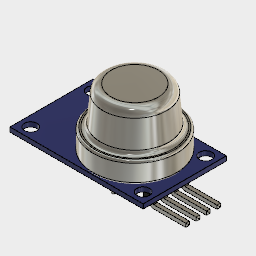
MQ135_sensor (Autodesk Fusion 360 design; units mm, degrees)
Autodesk Fusion 360 part; units mm, degrees
note: some values were not read from the file. Chosen so that the rebuilt part matches the saved one: which bodies a step acts on. Set by a fixed rule: which sketch regions a step uses.
sketch "Sketch1" plane through (0, 0, 0) normal (0, 0, 1) x (1, 0, 0)
  line L0 (-18.5, 15.5) -> (13.5, 15.5)
  line L1 (13.5, 15.5) -> (13.5, -4.5)
  line L2 (13.5, -4.5) -> (-18.5, -4.5)
  line L3 (-18.5, -4.5) -> (-18.5, 15.5)
  line L4 (-18.5, 5.5) -> (13.5, 5.5) construction
  line L5 (-2.5, 15.5) -> (-2.5, -4.5) construction
  line L6 (-16, 13) -> (11, 13) construction
  line L7 (11, 13) -> (11, -2) construction
  line L8 (11, -2) -> (-16, -2) construction
  line L9 (-16, -2) -> (-16, 13) construction
  circle A0 centre (-16, 13) radius 1.5
  circle A1 centre (-16, -2) radius 1.5
  circle A2 centre (11, 13) radius 1.5
  circle A3 centre (11, -2) radius 1.5
  line L10 (11.5, 19) -> (11.5, -9) construction
  circle A4 centre (1.5, 5.5) radius 10
  dimension "d1" = 20
  dimension "d2" = 32
  dimension "d3" = 27
  dimension "d4" = 15
  dimension "d5" = 3
  dimension "d6" = 3
  dimension "d7" = 3
  dimension "d8" = 3
  dimension "d9" = 2
  dimension "d10" = 20
  measures "d1" distance of L0.start L2.end
  measures "d2" distance of L0.start L0.end
  measures "d3" distance of L6.start L6.end
  measures "d4" distance of L6.start L8.end
  measures "d5" diameter of A0
  measures "d6" diameter of A1
  measures "d7" diameter of A2
  measures "d8" diameter of A3
  measures "d9" distance of L1 L10
  measures "d10" diameter of A4
extrude "Extrude1" add sketch "Sketch1" against normal blind 1.1 makes body 1
extrude "Extrude2" add sketch "Sketch1" along normal blind 5 separate body contours A4 makes body 2
sketch "Sketch2" plane through (0, 0, 5) normal (0, 0, 1) x (-1, 0, 0)
  circle A0 centre (-1.5, -5.5) radius 10
  circle A1 centre (-1.5, -5.5) radius 8.25
  dimension "d15" = 16.5
  measures "d15" diameter of A1
extrude "Extrude3" add sketch "Sketch2" along normal blind 9 draft -5 contours A1 bodies 2
fillet "Fillet1" radius 2 1 edges at (8.4576, 2.8014, 14) on bodies 2
fillet "Fillet2" radius 1 1 edges at (9.1917, 2.5167, 5) on bodies 2
fillet "Fillet3" radius 0.5 2 edges at (-7.8233, 1.8838, 5) (-7.8233, 1.8838, 0) on bodies 2
sketch "Sketch3" plane through (0, 0, -1.1) normal (0, 0, -1) x (1, 0, 0)
  circle A0 centre (11, 2) radius 1.5
  circle A1 centre (11, -13) radius 1.5
  circle A2 centre (-16, 2) radius 1.5
  circle A3 centre (-16, -13) radius 1.5
  line L0 (13.5, 4.5) -> (-18.5, 4.5)
  line L1 (-18.5, 4.5) -> (-18.5, -15.5)
  line L2 (-18.5, -15.5) -> (13.5, -15.5)
  line L3 (13.5, -15.5) -> (13.5, 4.5)
  line L4 (-12, -20) -> (-12, 7) construction
  line L5 (-18.5, 4.5) -> (-18.5, -15.5)
  line L6 (-12, -15) -> (-5, -15)
  line L7 (-5, -15) -> (-5, -8)
  line L8 (-5, -8) -> (-12, -8)
  line L9 (-12, -8) -> (-12, -15)
  line L10 (1.5, -19) -> (1.5, 10) construction
  line L11 (13.5, -15.5) -> (13.5, 4.5)
  circle A4 centre (1.5, -5.5) radius 5
  circle A5 centre (1.5, -10.5) radius 0.5
  circle A6 centre (5.0355, -9.0355) radius 0.5
  circle A7 centre (5.0355, -1.9645) radius 0.5
  circle A8 centre (1.5, -0.5) radius 0.5
  circle A9 centre (-2.0355, -1.9645) radius 0.5
  circle A10 centre (-2.0355, -9.0355) radius 0.5
  line L12 (11, -10.5) -> (8.5, -10.5)
  line L13 (8.5, -10.5) -> (8.5, -0.5)
  line L14 (8.5, -0.5) -> (11, -0.5)
  line L15 (11, -0.5) -> (11, -10.5)
  line L16 (11, -13) -> (11, 2)
  line L17 (-18.5, -5.5) -> (13.5, -5.5)
  point P0 (1.5, -5.5)
  dimension "d21" = 6.5
  dimension "d22" = 7
  dimension "d23" = 7
  dimension "d24" = 12
  dimension "d25" = 10
  dimension "d26" = 1
  dimension "d28" = 360
  dimension "d29" = 10
  dimension "d30" = 2.5
  measures "d21" distance of L4 L5
  measures "d22" distance of L6.start L8.end
  measures "d23" distance of L6.start L6.end
  measures "d24" distance of L10 L11
  measures "d25" diameter of A4
  measures "d26" diameter of A5
  measures "d29" distance of L12.start L14.end
  measures "d30" distance of L12.start L12.end
extrude "Extrude4" add sketch "Sketch3" along normal blind 5 separate body contours L6 L7 L8 L9 makes body 3
extrude "Extrude5" add sketch "Sketch3" along normal blind 5 separate body contours A4 A9 | A4 A9 | A4 A10 | A4 A10 | A4 A7 | A4 A7 | A4 A6 | A4 A6 | A4 A8 | A4 A8 | A4 A5 | A4 A5 makes body 4 at (-2.5349, 9.0106, -4.4333) makes body 5 at (5.533, 2.0142, -2.7667) makes body 6 at (1.9975, 10.4502, -4.4333) makes body 7 at (-1.538, 2.0142, -2.7667) makes body 8 at (1.9975, 0.5498, -2.7667) makes body 9 at (5.533, 8.9857, -4.4333)
combine "Combine1" operation add target body 9 tool bodies 8 7 6 5 4 makes body 10 at (-1.538, 2.0142, -2.7667) makes body 11 at (5.533, 2.0142, -2.7667) makes body 12 at (1.9975, 0.5498, -2.7667) makes body 13 at (1.9975, 10.4502, -4.4333) makes body 14 at (-2.5349, 9.0106, -4.4333)
extrude "Extrude6" add sketch "Sketch3" along normal blind 2.5 separate body contours L13 L14 L15 L16 L17 | L12 L13 L15 L16 L17 makes body 15
sketch "Sketch6" plane through (0, 0, -6.1) normal (0, 0, -1) x (1, 0, 0)
  line L0 (-12, -8) -> (-12, -15)
  line L1 (-12, -15) -> (-5, -15)
  line L2 (-5, -15) -> (-5, -8)
  line L3 (-5, -8) -> (-12, -8)
  circle A0 centre (-8.5, -11.5) radius 1.5
  dimension "d49" = 3
  measures "d49" diameter of A0
extrude "Extrude9" cut sketch "Sketch6" against normal blind 2 contours A0 bodies 3
extrude "Extrude10" add sketch "Sketch6" against normal blind 2 separate body contours A0 makes body 16
sketch "Sketch7" plane through (0, 0, -6.1) normal (0, 0, -1) x (1, 0, 0)
  circle A0 centre (-8.5, -11.5) radius 1.5
  line L0 (-8.5, -9.7842) -> (-8.5, -13.4) construction
  line L1 (-10.3039, -11.5) -> (-6.8, -11.5) construction
  line L2 (-8.8, -9.8) -> (-8.2, -9.8)
  line L3 (-8.2, -9.8) -> (-8.2, -13.2)
  line L4 (-8.2, -13.2) -> (-8.8, -13.2)
  line L5 (-8.8, -13.2) -> (-8.8, -9.8)
  line L6 (-10.3, -11.2) -> (-6.8, -11.2)
  line L7 (-6.8, -11.2) -> (-6.8, -11.8)
  line L8 (-6.8, -11.8) -> (-10.3, -11.8)
  line L9 (-10.3, -11.8) -> (-10.3, -11.2)
  line L10 (-9.2, -10.8) -> (-10.0318, -10.8)
  line L11 (-10.0318, -10.8) -> (-10.0318, -9.9522)
  line L12 (-10.0318, -9.9522) -> (-9.2, -9.9522)
  line L13 (-9.2, -9.9522) -> (-9.2, -10.8)
  line L14 (-9.2, -12.2) -> (-10.1, -12.2)
  line L15 (-10.1, -12.2) -> (-10.1, -13.1)
  line L16 (-10.1, -13.1) -> (-9.2, -13.1)
  line L17 (-9.2, -13.1) -> (-9.2, -12.2)
extrude "Extrude11" cut sketch "Sketch7" against normal blind 0.5 contours A0 L3 L6 L8 | A0 L3 L5 L6 | L3 L5 L6 L8 | A0 L3 L5 L8 | A0 L5 L6 L8 | A0 L10 L13 | A0 L14 L17 bodies 16
sketch "Sketch8" plane through (0, 0, -3.6) normal (0, 0, -1) x (1, 0, 0)
  line L0 (11, -10.5) -> (11, -0.5)
  line L1 (11, -0.5) -> (8.5, -0.5)
  line L2 (8.5, -0.5) -> (8.5, -10.5)
  line L3 (8.5, -10.5) -> (11, -10.5)
  line L4 (8.5, -5.5) -> (11, -5.5) construction
  line L5 (8.5, -0.5) -> (11, -0.5)
  line L6 (11, -0.5) -> (11, -5.5)
  line L7 (11, -5.5) -> (8.5, -5.5)
  line L8 (8.5, -5.5) -> (8.5, -0.5)
  line L9 (8.5, -3) -> (11, -3) construction
  line L10 (8.5, -5.5) -> (11, -5.5)
  line L11 (11, -5.5) -> (11, -10.5)
  line L12 (11, -10.5) -> (8.5, -10.5)
  line L13 (8.5, -10.5) -> (8.5, -5.5)
  line L14 (11, -8) -> (8.5, -8)
  line L15 (8.5, -0.5) -> (11, -0.5)
  line L16 (11, -0.5) -> (11, -3)
  line L17 (11, -3) -> (8.5, -3)
  line L18 (8.5, -3) -> (8.5, -0.5)
  line L19 (8.5, -3) -> (11, -3)
  line L20 (11, -3) -> (11, -5.5)
  line L21 (11, -5.5) -> (8.5, -5.5)
  line L22 (8.5, -5.5) -> (8.5, -3)
  line L23 (8.5, -5.5) -> (11, -5.5)
  line L24 (11, -5.5) -> (11, -8)
  line L25 (11, -8) -> (8.5, -8)
  line L26 (8.5, -8) -> (8.5, -5.5)
  line L27 (8.5, -8) -> (11, -8)
  line L28 (11, -8) -> (11, -10.5)
  line L29 (11, -10.5) -> (8.5, -10.5)
  line L30 (8.5, -10.5) -> (8.5, -8)
  line L31 (10.2, -2.1986) -> (9.3, -2.1986)
  line L32 (9.3, -2.1986) -> (9.3, -1.2986)
  line L33 (9.3, -1.2986) -> (10.2, -1.2986)
  line L34 (10.2, -1.2986) -> (10.2, -2.1986)
  line L35 (10.2, -2.1986) -> (9.3, -1.2986) construction
  line L36 (9.3, -2.1986) -> (10.2, -1.2986) construction
  line L37 (8.5, -4.25) -> (11, -4.25)
  line L38 (8.5, -6.75) -> (11, -6.75)
  line L39 (8.5, -9.25) -> (11, -9.25)
  line L40 (10.2, -4.7) -> (9.3, -4.7)
  line L41 (9.3, -4.7) -> (9.3, -3.8)
  line L42 (9.3, -3.8) -> (10.2, -3.8)
  line L43 (10.2, -3.8) -> (10.2, -4.7)
  line L44 (10.2, -4.7) -> (9.3, -3.8) construction
  line L45 (9.3, -4.7) -> (10.2, -3.8) construction
  line L46 (10.2, -7.2) -> (9.3, -7.2)
  line L47 (9.3, -7.2) -> (9.3, -6.3)
  line L48 (9.3, -6.3) -> (10.2, -6.3)
  line L49 (10.2, -6.3) -> (10.2, -7.2)
  line L50 (10.2, -7.2) -> (9.3, -6.3) construction
  line L51 (9.3, -7.2) -> (10.2, -6.3) construction
  line L52 (10.2, -9.7) -> (9.3, -9.7)
  line L53 (9.3, -9.7) -> (9.3, -8.8)
  line L54 (9.3, -8.8) -> (10.2, -8.8)
  line L55 (10.2, -8.8) -> (10.2, -9.7)
  line L56 (10.2, -9.7) -> (9.3, -8.8) construction
  line L57 (9.3, -9.7) -> (10.2, -8.8) construction
  point P0 (9.75, -1.7486)
  point P1 (9.75, -4.25)
  point P2 (9.75, -6.75)
  point P3 (9.75, -9.25)
  dimension "d56" = 0.9
  dimension "d57" = 0.9
  dimension "d58" = 0.9
  dimension "d59" = 0.9
  dimension "d60" = 0.9
  dimension "d61" = 0.9
  dimension "d62" = 0.9
  dimension "d63" = 0.9
  measures "d56" distance of L31.end L32.end
  measures "d57" distance of L32.end L33.end
  measures "d58" distance of L40.end L41.end
  measures "d59" distance of L41.end L42.end
  measures "d60" distance of L46.end L47.end
  measures "d61" distance of L47.end L48.end
  measures "d62" distance of L52.end L53.end
  measures "d63" distance of L53.end L54.end
extrude "Extrude12" add sketch "Sketch8" along normal blind 2 separate body contours L39 L52 L53 L55 | L39 L53 L54 L55 | L38 L46 L47 L49 | L38 L47 L48 L49 | L37 L40 L41 L43 | L37 L41 L42 L43 | L31 L32 L33 L34 makes body 17 at (9.3, 4.4, -4.2667) makes body 18 at (9.3, 6.9, -4.2667) makes body 19 at (9.3, 1.8986, -4.2667) makes body 20 at (10.2, 9.1, -4.2667)
sketch "Sketch9" plane through (10.2, 0, 0) normal (1, 0, 0) x (0, 1, 0)
  line L0 (9.7, -3.6) -> (8.8, -3.6)
  line L1 (8.8, -3.6) -> (8.8, -5.6)
  line L2 (8.8, -5.6) -> (9.7, -5.6)
  line L3 (9.7, -5.6) -> (9.7, -3.6)
  line L4 (1.2986, -5.6) -> (2.1986, -5.6)
  line L5 (2.1986, -5.6) -> (2.1986, -4.7)
  line L6 (2.1986, -4.7) -> (1.2986, -4.7)
  line L7 (1.2986, -4.7) -> (1.2986, -5.6)
  line L8 (3.8, -5.6) -> (4.7, -5.6)
  line L9 (4.7, -5.6) -> (4.7, -4.7)
  line L10 (4.7, -4.7) -> (3.8, -4.7)
  line L11 (3.8, -4.7) -> (3.8, -5.6)
  line L12 (4.7, -3.6) -> (4.7, -5.6)
  line L13 (6.3, -4.7) -> (7.2, -4.7)
  line L14 (7.2, -4.7) -> (7.2, -5.6)
  line L15 (7.2, -5.6) -> (6.3, -5.6)
  line L16 (6.3, -5.6) -> (6.3, -4.7)
  line L17 (6.3, -3.6) -> (6.3, -5.6)
  line L18 (8.8, -4.7) -> (9.7, -4.7)
  line L19 (9.7, -4.7) -> (9.7, -5.6)
  line L20 (9.7, -5.6) -> (8.8, -5.6)
  line L21 (8.8, -5.6) -> (8.8, -4.7)
  point P0 (1.2986, -5.6)
  point P1 (3.8, -5.6)
  point P2 (7.2, -5.6)
  dimension "d66" = 0.9
  dimension "d67" = 0.9
  measures "d66" distance of P0 L4.end
  measures "d67" distance of P0 L6.end
extrude "Extrude13" add sketch "Sketch9" along normal blind 8 contours L1 L2 L3 L18 L19 L20 L21 | L4 L5 L6 L7 | L8 L9 L10 L11 L12 | L13 L14 L15 L16 L17 bodies 17 18 19 20
fillet "Fillet4" radius 0.8 4 edges at (9.3, 4.25, -5.6) (9.3, 6.75, -5.6) (9.3, 1.7486, -5.6) (9.3, 9.25, -5.6) on bodies 17 18 19 20
chamfer "Chamfer1" distance 0.3 angle 45 16 edges at (18.2, 1.7486, -5.6) (18.2, 1.2986, -5.15) (18.2, 1.7486, -4.7) (18.2, 2.1986, -5.15) (18.2, 3.8, -5.15) (18.2, 4.25, -4.7) (18.2, 4.25, -5.6) (18.2, 4.7, -5.15) (18.2, 6.75, -4.7) (18.2, 6.75, -5.6) (18.2, 6.3, -5.15) (18.2, 7.2, -5.15) (18.2, 9.25, -4.7) (18.2, 9.7, -5.15) (18.2, 9.25, -5.6) (18.2, 8.8, -5.15) on bodies 17 18 19 20
